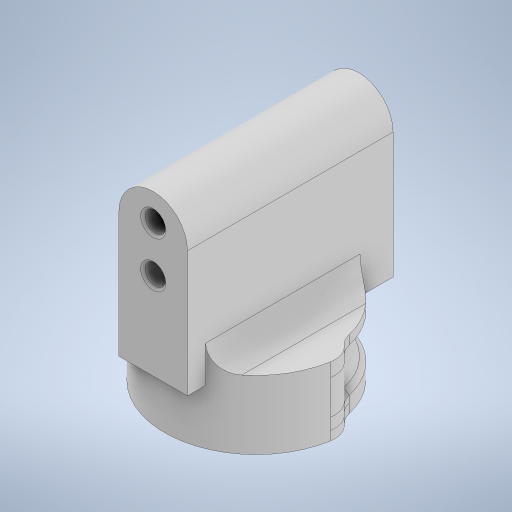
# Autodesk Inventor part: 회전 축 고정대
Saved by Autodesk Inventor 2023 (Build 270158000, 158)
## iProperties
Created: 2022-09-04
Part Number: 회전 축 고정대
Material: 일반
Document SubType Name: Modeling
Designer: fly01
Density: 1 g/cm^3
Appearance: 기본값
Author: fly01
Autodesk Inventor part; units mm, degrees
ref_plane "YZ Plane" through (0, 0, 0) normal (1, 0, 0) x (0, 1, 0)
ref_plane "XZ Plane" through (0, 0, 0) normal (0, 1, 0) x (-1, 0, 0)
ref_plane "XY Plane" through (0, 0, 0) normal (0, 0, 1) x (1, 0, 0)
sketch "스케치1" plane through (0, 0, 0) normal (0, 0, 1) x (1, 0, 0)
  line L0 (-7.5, -17.5) -> (7.5, -17.5)
  line L1 (7.5, -17.5) -> (7.5, 17.5)
  line L2 (7.5, 17.5) -> (-7.5, 17.5)
  line L3 (-7.5, 17.5) -> (-7.5, -17.5)
  line L4 (-7.5, -17.5) -> (7.5, 17.5) construction
  line L5 (7.5, -17.5) -> (-7.5, 17.5) construction
  point P0 (0, 0)
  dimension "d0" = 15
  dimension "d1" = 35
  constraints: 12 end point, 2 midpoint, 2 parallel, 1 horizontal, 1 perpendicular
  measures "d0" distance of L2.end L1.end
  measures "d1" distance of L1.end L0.end
extrude "돌출1" add sketch "스케치1" along normal mid plane 45
sketch "스케치2" plane through (0, 0, 22.5) normal (0, 0, 1) x (1, 0, 0)
  circle A0 centre (0, 11.5) radius 2.25
  circle A1 centre (0, 1.5) radius 2.25
  line L0 (-7.5, 17.5) -> (7.5, 17.5) projected
  point P0 (0, 0)
  point P1 (0, 17.5)
  point P2 (0, 17.5)
  dimension "d4" = 4.5
  dimension "d5" = 4.5
  dimension "d6" = 10
  dimension "d43" = 6
  constraints: 2 centre point, 2 midpoint, 2 vertical alignment
  measures "d4" diameter of A0
  measures "d5" diameter of A1
  measures "d6" distance of A0.centre A1.centre
  measures "d43" distance of point (0, 17.5) A0.centre
extrude "돌출2" cut sketch "스케치2" against normal up to surface (45 mm away)
fillet "모깎기1" radius 7.5 2 edges at (7.5, 17.5, 0) (-7.5, 17.5, 0)
chamfer "모따기1" distance 0.5 angle 45 4 edges at (-2.25, 11.5, 22.5) (-2.25, 1.5, 22.5) (-2.25, 1.5, -22.5) (-2.25, 11.5, -22.5)
sketch "스케치3" plane through (-7.5, -17.5, -22.5) normal (0, -1, 0) x (1, 0, 0)
  circle A0 centre (7.5, 22.5) radius 20
  line L0 (27.3997, 20.5) -> (-12.3997, 20.5)
  circle A1 centre (7.5, 22.5) radius 17
  point P0 (7.5, 22.5)
  point P1 (-9.3819, 20.5)
  point P2 (24.3819, 20.5)
  dimension "d14" = 40
  dimension "d15" = 2
  dimension "d16" = 3
  constraints: 2 centre point, 2 end point, 2 point on circle, 1 coincident, 1 horizontal
  measures "d14" diameter of A0
  measures "d15" distance from line of A1.centre L0
  measures "d16" radial gap between concentric circles of A0 A1
extrude "돌출3" add sketch "스케치3" along normal blind 10 contours A0 L0 A1 | A1 L0 | L0 A1 picked at (26.1409, 25.4527)
extrude "돌출5" cut sketch "스케치3" along normal blind 7.5 contours A1 L0 | L0 A1
extrude "돌출6" add sketch "스케치3" against normal blind 3 contours A0 L0 A1 | A1 L0 | L0 A1 picked at (26.1409, 25.4527)
fillet "모깎기4" radius 5 6 edges at (19.8997, -21, -2) (-19.8997, -21, -2) (-16.8819, -16, -2) (-16.8819, -26.25, -2) (16.8819, -16, -2) (16.8819, -26.25, -2)
sketch "스케치5" plane through (-7.5, -27.5, -22.5) normal (0, -1, 0) x (1, 0, 0)
  arc A0 (24.069, 18.6964) -> (-9.069, 18.6964) centre (7.5, 22.5) ccw projected
  circle A1 centre (7.5, 22.5) radius 1.75
  point P0 (7.5, 22.5)
  dimension "d28" = 3.5
  constraints: 1 centre point, 1 coincident
  measures "d28" diameter of A1
extrude "돌출7" cut sketch "스케치5" against normal up to surface (10 mm away)
sketch "스케치6" plane through (-7.5, -27.5, -22.5) normal (0, -1, 0) x (1, 0, 0)
  circle A0 centre (7.5, 22.5) radius 1.75 projected
  circle A1 centre (7.5, 22.5) radius 1.5
  point P0 (7.5, 22.5)
  dimension "d31" = 3
  constraints: 1 centre point, 1 coincident
  measures "d31" diameter of A1
extrude "돌출8" cut sketch "스케치6" against normal blind 20 contours A1
chamfer "모따기2" distance 1 angle 45 7 edges at (0, -25, -17) (17.1381, -25, -2.3779) (-17.1381, -25, -2.3779) (13.3274, -17.5, -10.5537) (-13.3274, -17.5, -10.5537) (17.1381, -17.5, -2.3779) (-17.1381, -17.5, -2.3779)
fillet "모깎기5" radius 5 2 edges at (7.5, -14.5, 1.6422) (-7.5, -14.5, 1.6422)
sketch "스케치8" plane through (0, 0, -22.5) normal (0, 0, -1) x (-1, 0, 0)
  circle A0 centre (0, -8.5) radius 5.25
  circle A1 centre (0, 1.5) radius 2.75 projected
  point P0 (0, 0)
  dimension "d44" = 10.5
  dimension "d45" = 10
  constraints: 1 centre point
  measures "d44" diameter of A0
  measures "d45" distance of A0.centre A1.centre
extrude "돌출11" cut sketch "스케치8" against normal blind 5 contours A0
sketch "스케치9" plane through (-7.5, -27.5, -22.5) normal (0, -1, 0) x (1, 0, 0)
  circle A0 centre (7.5, 22.5) radius 1.75 projected
  spline S0 degree 2 poles (27.2115, 25.8846) (27.6805, 23.1533) (25.613, 21.308) knots 0 0 0 1 1 1 weights 1 0.874643 1 projected
  arc A1 (27.2115, 25.8846) -> (-12.2115, 25.8846) centre (7.5, 22.5) ccw projected
  spline S1 degree 2 poles (-10.613, 21.308) (-12.6805, 23.1533) (-12.2115, 25.8846) knots 0 0 0 1 1 1 weights 1 0.874643 1 projected
  spline S2 degree 2 poles (-9.069, 18.6964) (-9.4252, 20.248) (-10.613, 21.308) knots 0 0 0 1 1 1 weights 1 0.952866 1 projected
  arc A2 (-9.069, 18.6964) -> (24.069, 18.6964) centre (7.5, 22.5) ccw projected
  spline S3 degree 2 poles (25.613, 21.308) (24.4252, 20.248) (24.069, 18.6964) knots 0 0 0 1 1 1 weights 1 0.952866 1 projected
  point P0 (7.5, 22.5)
  constraints: 4 other
extrude "돌출12" add sketch "스케치9" along normal blind 2
sketch "스케치10" plane through (-7.5, -29.5, -22.5) normal (0, -1, 0) x (1, 0, 0)
  circle A0 centre (7.5, 22.5) radius 3.25
  dimension "d50" = 6.5
  constraints: 1 centre point, 1 coincident
  measures "d50" diameter of A0
extrude "돌출13" cut sketch "스케치10" against normal blind 3
